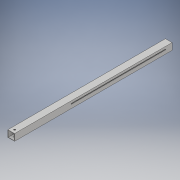
# Autodesk Inventor part: ScissorLiftBase
Saved by Autodesk Inventor 2018.3 (Build 223284000, 284)
## iProperties
Created: 2020-01-24
Part Number: ScissorLiftBase
Material: Generic
Document SubType Name: Modeling
Designer: Cooper
Density: 1 g/cm^3
Appearance: Default
Author: Cooper
Autodesk Inventor part; units mm, degrees
ref_plane "YZ Plane" through (0, 0, 0) normal (1, 0, 0) x (0, 1, 0)
ref_plane "XZ Plane" through (0, 0, 0) normal (0, 1, 0) x (-1, 0, 0)
ref_plane "XY Plane" through (0, 0, 0) normal (0, 0, 1) x (1, 0, 0)
sketch "Sketch1" plane through (0, 0, 0) normal (0, 0, 1) x (1, 0, 0)
  line L0 (0, 0) -> (25.4, 0)
  line L1 (25.4, 0) -> (25.4, 25.4)
  line L2 (25.4, 25.4) -> (0, 25.4)
  line L3 (0, 25.4) -> (0, 0)
  line L4 (1.5875, 23.8125) -> (23.8125, 23.8125)
  line L5 (23.8125, 23.8125) -> (23.8125, 1.5875)
  line L6 (23.8125, 1.5875) -> (1.5875, 1.5875)
  line L7 (1.5875, 1.5875) -> (1.5875, 23.8125)
  dimension "d0" = 25.4
  dimension "d1" = 25.4
  dimension "d2" = 1.5875
  constraints: 16 end point, 4 parallel, 2 perpendicular, 1 horizontal, 3 other
  measures "d0" distance of L2.end L0.start
  measures "d1" distance of L0.start L0.end
  measures "d2" distance between parallel lines of L2 L4
extrude "Extrusion1" add sketch "Sketch1" along normal blind 596.9
sketch "Sketch2" plane through (0, 0, 0) normal (-1, 0, 0) x (0, 0, 1)
  line L0 (0, 25.4) -> (0, 0) projected
  line L1 (0, 0) -> (596.9, 0) projected
  line L2 (596.9, 25.4) -> (596.9, 0) projected
  line L3 (0, 25.4) -> (596.9, 25.4) projected
  line L4 (25.4, 16.8275) -> (381, 16.8275)
  arc A0 (381, 13.6525) -> (381, 16.8275) centre (381, 15.24) ccw
  line L5 (381, 13.6525) -> (25.4, 13.6525)
  arc A1 (25.4, 16.8275) -> (25.4, 13.6525) centre (25.4, 15.24) ccw
  dimension "d5" = 3.175
  dimension "d6" = 355.6
  dimension "d9" = 10.16
  dimension "d24" = 25.4
  constraints: 4 end point, 4 point on circle, 4 tangent, 2 centre point, 1 horizontal, 1 parallel
  measures "d5" distance between parallel lines of L5 L4
  measures "d6" distance of A0.centre A1.centre
  measures "d9" distance from line of L3 A1.centre
  measures "d24" distance from line of L0 A1.centre
extrude "Extrusion2" cut sketch "Sketch2" against normal through all contours L4 A0 L5 A1
sketch "Sketch3" plane through (0, 25.4, 0) normal (0, 1, 0) x (1, 0, 0)
  line L0 (25.4, 0) -> (0, 0) projected
  line L1 (0, 0) -> (0, -596.9) projected
  line L2 (25.4, -596.9) -> (0, -596.9) projected
  line L3 (25.4, 0) -> (25.4, -596.9) projected
  point P0 (0, 0)
  point P1 (12.7, -584.2)
  dimension "d13" = 12.7
  dimension "d14" = 12.7
  dimension "d23" = 12.7
  measures "d13" distance from line of L1 point (12.7, -584.2)
  measures "d14" distance from line of L3 point (12.7, -584.2)
  measures "d23" distance from line of L2 point (12.7, -584.2)
hole "Hole1" at (12.7, 25.4, 584.2) direction (0, -1, 0) diameter 6.35 end through all
equation "\"d13\" = d14"
body "Solid1"
